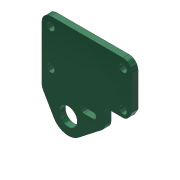
# Autodesk Inventor part: COXA_YAW_SERVO_FRONT
Saved by Autodesk Inventor 2019.4 (Build 234330000, 330)
## iProperties
Created: 2019-11-09
Part Number: COXA_YAW_SERVO_FRONT
Material: 一般
Document SubType Name: Modeling
Designer: y6tada
Density: 1 g/cm^3
Appearance: 滑らか - 濃い海緑
Author: y6tada
Autodesk Inventor part; units mm, degrees
ref_plane "YZ Plane" through (0, 0, 0) normal (1, 0, 0) x (0, 1, 0)
ref_plane "XZ Plane" through (0, 0, 0) normal (0, 1, 0) x (-1, 0, 0)
ref_plane "XY Plane" through (0, 0, 0) normal (0, 0, 1) x (1, 0, 0)
sketch "スケッチ1" plane through (0, 0, 0) normal (0, 0, 1) x (1, 0, 0)
  circle A0 centre (29.25, -6) radius 1.25 construction
  circle A1 centre (29.25, 6) radius 1.25 construction
  circle A2 centre (5.25, 6) radius 1.25 construction
  circle A3 centre (5.25, -6) radius 1.25 construction
  line L0 (42.5, -8.25) -> (0, -8.25) construction
  circle A4 centre (11.0231, -17.0183) radius 3 projected
  arc A5 (6.26, -19.7683) -> (16.5231, -17.0183) centre (11.0231, -17.0183) ccw construction
  line L1 (29.25, -8.25) -> (24.25, -8.25)
  line L2 (2.25, -12.019) -> (2.25, 6)
  line L3 (5.25, 9) -> (29.25, 9)
  arc A6 (6.26, -19.7683) -> (14.401, -21.3588) centre (11.0231, -17.0183) ccw
  arc A7 (2.25, -12.019) -> (2.6519, -13.519) centre (5.25, -12.019) ccw construction
  line L4 (6.26, -19.7683) -> (2.6519, -13.519)
  arc A8 (2.25, -12.019) -> (2.6519, -13.519) centre (5.25, -12.019) ccw
  arc A9 (5.25, 9) -> (2.25, 6) centre (5.25, 6) ccw
  arc A10 (32.25, 6) -> (29.25, 9) centre (29.25, 6) ccw
  arc A11 (29.25, -8.25) -> (31.1986, -7.125) centre (29.25, -6) ccw
  line L5 (31.1986, -7.125) -> (32.25, -5.3038)
  line L6 (32.25, -5.3038) -> (32.25, 6)
  line L7 (14.401, -21.3588) -> (22.2854, -15.223)
  line L8 (23.25, -13.25) -> (23.25, -9.25)
  arc A12 (24.25, -8.25) -> (23.25, -9.25) centre (24.25, -9.25) ccw
  arc A13 (22.2854, -15.223) -> (23.25, -13.25) centre (20.75, -13.25) ccw
  line L9 (33.25, 455.3781) -> (33.25, -190.243) construction
  line L10 (19.25, -13.55) -> (16.25, -13.55) construction
  line L11 (16.25, -13.55) -> (16.25, -11.55) construction
  line L12 (16.25, -11.55) -> (19.25, -11.55) construction
  line L13 (19.25, -11.55) -> (19.25, -13.55) construction
  line L14 (-2, -11.55) -> (-2, -13.55) construction
  line L15 (-2, -12.55) -> (28.8527, -12.55) construction
  line L16 (16.2, -13.6) -> (19.3, -13.6)
  line L17 (19.3, -13.6) -> (19.3, -11.5) construction
  line L18 (19.3, -11.5) -> (16.2, -11.5)
  line L19 (16.2, -11.5) -> (16.2, -13.6) construction
  arc A14 (19.3, -13.6) -> (19.3, -11.5) centre (19.3, -12.55) ccw
  arc A15 (16.2, -11.5) -> (16.2, -13.6) centre (16.2, -12.55) ccw
  point P0 (0, 0)
  point P1 (2.25, -8.25)
  dimension "d4" = 30
  dimension "d5" = 1
  dimension "d6" = 2.5
  dimension "d7" = 10
  dimension "d8" = 5
  dimension "d18" = 2
  dimension "d19" = 4
  dimension "d20" = 3
  dimension "d21" = 0.05
  constraints: 38 end point, 18 point on circle, 18 tangent, 9 centre point, 6 concentric, 5 coincident, 5 parallel, 4 perpendicular, 3 horizontal, 3 vertical, 2 point on line, 1 collinear, 1 midpoint, 8 other
  measures "d4" angle of L6 L5
  measures "d5" radius of A12
  measures "d6" radius of A13
  measures "d7" distance between parallel lines of L8 L9
  measures "d8" distance from line of L0 A13.centre
  measures "d18" distance of L10.end L11.end
  measures "d19" distance between parallel lines of L13 L8
  measures "d20" distance of L10.start L10.end
  measures "d21" distance between parallel lines of L10 L16
extrude "押し出し1" add sketch "スケッチ1" along normal blind 2
hole "穴1" at (5.25, -6, 0) at (5.25, 6, 0) at (29.25, 6, 0) at (29.25, -6, 0) direction (0, 0, 1) diameter 2.5 end through all
